Autodesk Fusion 360 part; units mm, degrees
(part 10 of 24)
  arc A1593 (61.7791, 45.6255) -> (62.0966, 45.6255) centre (61.9379, 45.6255) ccw
  arc A1594 (67.3925, 42.1213) -> (67.71, 42.1213) centre (67.5513, 42.1213) ccw
  arc A1595 (61.9357, 46.3347) -> (61.6424, 46.2132) centre (61.7891, 46.2739) ccw
  arc A1596 (63.9119, 46.0318) -> (63.7904, 45.7384) centre (63.8512, 45.8851) ccw
  line L433 (65.0555, 45.2726) -> (64.9496, 45.1667)
  arc A1597 (66.04, 45.4723) -> (66.04, 45.7898) centre (66.04, 45.6311) ccw
  line L434 (63.8511, 45.8851) -> (63.1489, 45.8851)
  line L435 (67.0245, 45.2726) -> (66.8321, 45.4124)
  line L436 (60.2439, 47.819) -> (59.8845, 47.9679)
  line L437 (66.04, 43.18) -> (67.5513, 43.18)
  arc A1598 (64.8373, 45.279) -> (65.0619, 45.0544) centre (64.9496, 45.1667) ccw
  line L438 (63.1489, 45.8851) -> (62.5, 45.6163)
  arc A1599 (65.6613, 45.7507) -> (65.7109, 45.4371) centre (65.6861, 45.5939) ccw
  arc A1600 (64.4392, 45.4697) -> (64.5607, 45.763) centre (64.4999, 45.6163) ccw
  arc A1601 (66.04, 43.3388) -> (66.04, 43.0213) centre (66.04, 43.1801) ccw
  line L439 (67.4406, 41.6601) -> (67.5141, 41.8863)
  arc A1602 (67.3573, 41.9111) -> (67.6709, 41.8615) centre (67.5141, 41.8863) ccw
  line L440 (67.5513, 42.1213) -> (67.5513, 43.18)
  line L441 (67.1928, 45.1043) -> (67.0245, 45.2726)
  line L442 (61.789, 46.2739) -> (60.519, 47.5439)
  arc A1603 (60.4068, 47.4317) -> (60.6313, 47.6562) centre (60.5191, 47.544) ccw
  arc A1604 (64.8373, 45.0544) -> (65.0619, 45.279) centre (64.9496, 45.1667) ccw
  arc A1605 (60.3562, 47.9313) -> (60.1317, 47.7068) centre (60.2439, 47.8191) ccw
  line L443 (65.2479, 45.4124) -> (65.0555, 45.2726)
  line L444 (64.9496, 45.1667) -> (64.5, 45.6163)
  arc A1606 (65.5319, 45.3789) -> (65.3878, 45.6618) centre (65.4599, 45.5204) ccw
  line L445 (67.0245, 41.0874) -> (67.1928, 41.2557)
  arc A1607 (66.5481, 40.9811) -> (66.6922, 40.6982) centre (66.6202, 40.8396) ccw
  arc A1608 (62.0966, 45.9145) -> (61.7791, 45.9145) centre (61.9379, 45.9145) ccw
  arc A1609 (67.3212, 45.1977) -> (67.0643, 45.011) centre (67.1928, 45.1044) ccw
  arc A1610 (59.9453, 48.1146) -> (59.8238, 47.8212) centre (59.8846, 47.9679) ccw
  line L446 (59.8845, 47.9679) -> (59.2617, 47.9679)
  arc A1611 (66.6922, 45.6618) -> (66.5481, 45.3789) centre (66.6201, 45.5204) ccw
  arc A1612 (60.1832, 47.6724) -> (60.3047, 47.9657) centre (60.2439, 47.8191) ccw
  arc A1613 (65.8813, 43.18) -> (66.1988, 43.18) centre (66.0401, 43.18) ccw
  arc A1614 (65.1677, 45.1603) -> (64.9432, 45.3848) centre (65.0555, 45.2726) ccw
  line L447 (60.519, 47.5439) -> (60.2439, 47.819)
  arc A1615 (61.8992, 45.4697) -> (62.0207, 45.763) centre (61.96, 45.6163) ccw
  line L448 (62.23, 45.3463) -> (61.96, 45.6163)
  arc A1616 (62.4393, 45.763) -> (62.5608, 45.4697) centre (62.5001, 45.6164) ccw
  line L449 (65.4599, 45.5204) -> (65.2479, 45.4124)
  arc A1617 (65.4108, 45.6714) -> (65.5089, 45.3694) centre (65.4598, 45.5204) ccw
  arc A1618 (61.7912, 45.8538) -> (62.0846, 45.9753) centre (61.9379, 45.9145) ccw
  arc A1619 (67.7081, 42.0964) -> (67.3945, 42.1461) centre (67.5513, 42.1212) ccw
  arc A1620 (64.9621, 45.401) -> (65.1488, 45.1441) centre (65.0555, 45.2726) ccw
  arc A1621 (67.3631, 44.4246) -> (67.6651, 44.5228) centre (67.5141, 44.4737) ccw
  line L450 (66.8321, 40.9476) -> (67.0245, 41.0874)
  arc A1622 (66.04, 43.0213) -> (66.04, 43.3388) centre (66.04, 43.1801) ccw
  arc A1623 (65.1758, 45.5538) -> (65.32, 45.2709) centre (65.2479, 45.4124) ccw
  line L451 (65.6861, 45.5939) -> (65.4599, 45.5204)
  arc A1624 (67.1368, 45.3848) -> (66.9123, 45.1603) centre (67.0246, 45.2726) ccw
  arc A1625 (63.8511, 45.7263) -> (63.8511, 46.0438) centre (63.8511, 45.8851) ccw
  arc A1626 (67.5513, 43.0212) -> (67.5513, 43.3387) centre (67.5513, 43.18) ccw
  arc A1627 (66.1987, 45.6311) -> (65.8812, 45.6311) centre (66.04, 45.6311) ccw
  line L452 (60.6089, 47.7647) -> (61.3111, 47.7647)
  arc A1628 (62.872, 49.1181) -> (62.5786, 49.2396) centre (62.7253, 49.1788) ccw
  line L453 (61.9379, 45.6255) -> (61.9379, 45.9145)
  line L454 (61.9379, 45.9145) -> (61.789, 46.2739)
  arc A1629 (65.8812, 43.18) -> (66.1987, 43.18) centre (66.04, 43.18) ccw
  line L455 (66.04, 45.6311) -> (65.9211, 45.6311)
  arc A1630 (58.8319, 51.442) -> (58.7104, 51.1486) centre (58.7711, 51.2953) ccw
  arc A1631 (57.3593, 51.1732) -> (57.4808, 50.8799) centre (57.42, 51.0266) ccw
  line L456 (61.3111, 51.2953) -> (60.6089, 51.2953)
  line L457 (61.3111, 47.7647) -> (61.96, 48.0335)
  arc A1632 (61.8477, 48.1457) -> (62.0722, 47.9212) centre (61.9599, 48.0335) ccw
  arc A1633 (62.5786, 49.8204) -> (62.872, 49.9419) centre (62.7253, 49.8812) ccw
  arc A1634 (65.7352, 45.4429) -> (65.637, 45.7449) centre (65.6861, 45.5939) ccw
  arc A1635 (59.5777, 50.8688) -> (59.8023, 50.6443) centre (59.69, 50.7566) ccw
  arc A1636 (62.0207, 47.8868) -> (61.8992, 48.1801) centre (61.9599, 48.0334) ccw
  arc A1637 (62.6032, 50.5907) -> (62.3099, 50.4692) centre (62.4566, 50.5299) ccw
  line L458 (61.96, 48.0335) -> (62.4565, 48.53)
  line L459 (66.04, 45.6311) -> (66.04, 43.18)
  arc A1638 (65.3412, 45.2839) -> (65.1546, 45.5408) centre (65.2479, 45.4124) ccw
  line L460 (57.15, 50.7565) -> (56.88, 51.0265)
  arc A1639 (62.5665, 49.1789) -> (62.884, 49.1789) centre (62.7253, 49.1789) ccw
  arc A1640 (60.0208, 48.1801) -> (59.8993, 47.8868) centre (59.96, 48.0335) ccw
  arc A1641 (59.8023, 48.1912) -> (59.5777, 48.4157) centre (59.69, 48.3035) ccw
  line L461 (59.2617, 47.9679) -> (59.42, 48.0335)
  arc A1642 (62.0722, 45.7286) -> (61.8477, 45.5041) centre (61.9599, 45.6164) ccw
  line L462 (61.96, 45.6163) -> (61.9379, 45.6255)
  line L463 (66.04, 43.18) -> (66.04, 45.6311)
  arc A1643 (59.5322, 51.1388) -> (59.3077, 50.9143) centre (59.42, 51.0266) ccw
  arc A1644 (59.8478, 47.9212) -> (60.0723, 48.1457) centre (59.9601, 48.0334) ccw
  arc A1645 (60.6313, 47.6562) -> (60.4068, 47.4317) centre (60.5191, 47.5439) ccw
  arc A1646 (59.3077, 48.1457) -> (59.5322, 47.9212) centre (59.42, 48.0335) ccw
  arc A1647 (62.1177, 45.2341) -> (62.3423, 45.4586) centre (62.23, 45.3464) ccw
  arc A1648 (61.6768, 46.1617) -> (61.9013, 46.3862) centre (61.7891, 46.2739) ccw
  arc A1649 (60.6089, 47.9235) -> (60.6089, 47.606) centre (60.6089, 47.7648) ccw
  line L464 (58.7711, 51.2953) -> (58.0689, 51.2953)
  arc A1650 (57.5323, 50.9143) -> (57.3078, 51.1388) centre (57.4201, 51.0266) ccw
  line L465 (62.5, 45.6163) -> (62.23, 45.3463)
  arc A1651 (65.9211, 45.7898) -> (65.9211, 45.4723) centre (65.9211, 45.6311) ccw
  arc A1652 (59.8845, 47.8091) -> (59.8845, 48.1266) centre (59.8845, 47.9679) ccw
  arc A1653 (59.3592, 50.8799) -> (59.4807, 51.1732) centre (59.42, 51.0266) ccw
  arc A1654 (58.1296, 51.1486) -> (58.0081, 51.442) centre (58.0689, 51.2953) ccw
  arc A1655 (62.0722, 51.1388) -> (61.8477, 50.9143) centre (61.9599, 51.0266) ccw
  arc A1656 (66.1589, 45.4723) -> (66.1589, 45.7898) centre (66.1589, 45.6311) ccw
  line L466 (59.69, 50.7565) -> (59.42, 51.0265)
  line L467 (62.7253, 49.1789) -> (62.7253, 49.8811)
  arc A1657 (56.9922, 51.1388) -> (56.7677, 50.9143) centre (56.88, 51.0266) ccw
  arc A1658 (63.2096, 45.7384) -> (63.0881, 46.0318) centre (63.1488, 45.8851) ccw
  arc A1659 (60.5481, 47.618) -> (60.6696, 47.9114) centre (60.6089, 47.7647) ccw
  arc A1660 (64.6122, 45.7286) -> (64.3877, 45.5041) centre (64.4999, 45.6163) ccw
  arc A1661 (62.5688, 48.4178) -> (62.3443, 48.6423) centre (62.4565, 48.53) ccw
  arc A1662 (62.1177, 45.4586) -> (62.3423, 45.2341) centre (62.23, 45.3464) ccw
  arc A1663 (65.8813, 43.18) -> (66.1988, 43.18) centre (66.0401, 43.18) ccw
  line L468 (57.42, 51.0265) -> (57.15, 50.7565)
  arc A1664 (57.0377, 50.8688) -> (57.2623, 50.6443) centre (57.15, 50.7566) ccw
  arc A1665 (66.04, 43.3388) -> (66.04, 43.0213) centre (66.04, 43.1801) ccw
  arc A1666 (61.3111, 51.1365) -> (61.3111, 51.454) centre (61.3111, 51.2953) ccw
  arc A1667 (61.2504, 47.9114) -> (61.3719, 47.618) centre (61.3111, 47.7647) ccw
  line L469 (62.4565, 50.53) -> (61.96, 51.0265)
  arc A1668 (59.5777, 50.6443) -> (59.8023, 50.8688) centre (59.69, 50.7566) ccw
  line L470 (62.7253, 49.8811) -> (62.4565, 50.53)
  arc A1669 (60.6089, 51.454) -> (60.6089, 51.1365) centre (60.6089, 51.2953) ccw
  arc A1670 (58.0689, 51.454) -> (58.0689, 51.1365) centre (58.0689, 51.2953) ccw
  line L471 (58.0689, 51.2953) -> (57.42, 51.0265)
  line L472 (59.42, 48.0335) -> (59.69, 48.3035)
  line L473 (51.1511, 51.2953) -> (50.4489, 51.2953)
  arc A1671 (57.0377, 50.6443) -> (57.2623, 50.8688) centre (57.15, 50.7566) ccw
  arc A1672 (49.7393, 51.1732) -> (49.8608, 50.8799) centre (49.8, 51.0266) ccw
  arc A1673 (49.1992, 50.8799) -> (49.3207, 51.1732) centre (49.26, 51.0266) ccw
  arc A1674 (52.9889, 51.454) -> (52.9889, 51.1365) centre (52.9889, 51.2953) ccw
  line L474 (59.96, 51.0265) -> (59.69, 50.7565)
  arc A1675 (52.4523, 50.9143) -> (52.2278, 51.1388) centre (52.34, 51.0266) ccw
  arc A1676 (61.3111, 47.606) -> (61.3111, 47.9235) centre (61.3111, 47.7648) ccw
  arc A1677 (59.2617, 48.1266) -> (59.2617, 47.8091) centre (59.2617, 47.9679) ccw
  arc A1678 (59.4807, 47.8868) -> (59.3592, 48.1801) centre (59.42, 48.0335) ccw
  arc A1679 (59.8993, 51.1732) -> (60.0208, 50.8799) centre (59.9601, 51.0266) ccw
  line L475 (59.96, 48.0335) -> (60.6089, 47.7647)
  arc A1680 (61.8992, 50.8799) -> (62.0207, 51.1732) centre (61.9599, 51.0266) ccw
  line L476 (59.42, 51.0265) -> (58.7711, 51.2953)
  line L477 (52.9889, 51.2953) -> (52.34, 51.0265)
  line L478 (49.8, 51.0265) -> (49.53, 50.7565)
  line L479 (61.96, 51.0265) -> (61.3111, 51.2953)
  arc A1681 (47.9089, 51.454) -> (47.9089, 51.1365) centre (47.9089, 51.2953) ccw
  arc A1682 (55.5289, 51.454) -> (55.5289, 51.1365) centre (55.5289, 51.2953) ccw
  arc A1683 (62.884, 49.8811) -> (62.5665, 49.8811) centre (62.7253, 49.8811) ccw
  arc A1684 (51.9122, 51.1388) -> (51.6877, 50.9143) centre (51.7999, 51.0266) ccw
  line L480 (54.34, 51.0265) -> (53.6911, 51.2953)
  arc A1685 (54.2792, 50.8799) -> (54.4007, 51.1732) centre (54.34, 51.0266) ccw
  arc A1686 (61.3719, 51.442) -> (61.2504, 51.1486) centre (61.3112, 51.2953) ccw
  line L481 (60.6089, 51.2953) -> (59.96, 51.0265)
  arc A1687 (46.8322, 51.1388) -> (46.6077, 50.9143) centre (46.72, 51.0266) ccw
  arc A1688 (54.4977, 50.8688) -> (54.7223, 50.6443) centre (54.61, 50.7566) ccw
  arc A1689 (51.1511, 51.1365) -> (51.1511, 51.454) centre (51.1511, 51.2953) ccw
  arc A1690 (52.2793, 51.1732) -> (52.4008, 50.8799) centre (52.3401, 51.0266) ccw
  line L482 (56.2311, 51.2953) -> (55.5289, 51.2953)
  line L483 (54.61, 50.7565) -> (54.34, 51.0265)
  arc A1691 (46.6592, 50.8799) -> (46.7807, 51.1732) centre (46.72, 51.0265) ccw
  arc A1692 (47.3723, 50.9143) -> (47.1478, 51.1388) centre (47.2601, 51.0266) ccw
  line L484 (51.8, 51.0265) -> (51.1511, 51.2953)
  arc A1693 (54.4522, 51.1388) -> (54.2277, 50.9143) centre (54.3399, 51.0266) ccw
  line L485 (50.4489, 51.2953) -> (49.8, 51.0265)
  arc A1694 (46.8777, 50.8688) -> (47.1023, 50.6443) centre (46.99, 50.7566) ccw
  arc A1695 (46.8777, 50.6443) -> (47.1023, 50.8688) centre (46.99, 50.7566) ccw
  arc A1696 (56.2919, 51.442) -> (56.1704, 51.1486) centre (56.2311, 51.2953) ccw
  line L486 (59.69, 48.3035) -> (59.96, 48.0335)
  arc A1697 (59.2009, 48.1146) -> (59.3224, 47.8212) centre (59.2616, 47.9679) ccw
  arc A1698 (58.7711, 51.1365) -> (58.7711, 51.454) centre (58.7711, 51.2953) ccw
  line L487 (49.53, 50.7565) -> (49.26, 51.0265)
  line L488 (46.72, 51.0265) -> (46.0711, 51.2953)
  line L489 (49.26, 51.0265) -> (48.6111, 51.2953)
  arc A1699 (54.4977, 50.6443) -> (54.7223, 50.8688) centre (54.61, 50.7566) ccw
  arc A1700 (60.0723, 50.9143) -> (59.8478, 51.1388) centre (59.9601, 51.0266) ccw
  line L490 (53.6911, 51.2953) -> (52.9889, 51.2953)
  arc A1701 (62.3099, 48.5908) -> (62.6032, 48.4693) centre (62.4566, 48.5301) ccw
  arc A1702 (54.8193, 51.1732) -> (54.9408, 50.8799) centre (54.8801, 51.0266) ccw
  arc A1703 (46.1319, 51.442) -> (46.0104, 51.1486) centre (46.0712, 51.2953) ccw
  arc A1704 (56.2311, 51.1365) -> (56.2311, 51.454) centre (56.2311, 51.2953) ccw
  line L491 (62.4565, 48.53) -> (62.7253, 49.1789)
  arc A1705 (54.9923, 50.9143) -> (54.7678, 51.1388) centre (54.8801, 51.0266) ccw
  arc A1706 (62.3443, 50.4177) -> (62.5688, 50.6422) centre (62.4566, 50.53) ccw
  line L492 (46.99, 50.7565) -> (46.72, 51.0265)
  line L493 (47.9089, 51.2953) -> (47.26, 51.0265)
  arc A1707 (55.5896, 51.1486) -> (55.4681, 51.442) centre (55.5289, 51.2953) ccw
  arc A1708 (51.2119, 51.442) -> (51.0904, 51.1486) centre (51.1512, 51.2953) ccw
  arc A1709 (50.4489, 51.454) -> (50.4489, 51.1365) centre (50.4489, 51.2953) ccw
  arc A1710 (60.6696, 51.1486) -> (60.5481, 51.442) centre (60.6089, 51.2953) ccw
  arc A1711 (59.8023, 48.4157) -> (59.5777, 48.1912) centre (59.69, 48.3035) ccw
  arc A1712 (51.9577, 50.6443) -> (52.1823, 50.8688) centre (52.07, 50.7566) ccw
  arc A1713 (53.7519, 51.442) -> (53.6304, 51.1486) centre (53.6912, 51.2953) ccw
  arc A1714 (42.2923, 50.9143) -> (42.0678, 51.1388) centre (42.18, 51.0266) ccw
  line L494 (54.88, 51.0265) -> (54.61, 50.7565)
  arc A1715 (47.1993, 51.1732) -> (47.3208, 50.8799) centre (47.26, 51.0266) ccw
  arc A1716 (41.7977, 50.6443) -> (42.0223, 50.8688) centre (41.91, 50.7566) ccw
  arc A1717 (53.6911, 51.1365) -> (53.6911, 51.454) centre (53.6911, 51.2953) ccw
  line L495 (47.26, 51.0265) -> (46.99, 50.7565)
  arc A1718 (49.4177, 50.6443) -> (49.6423, 50.8688) centre (49.53, 50.7566) ccw
  line L496 (45.3689, 51.2953) -> (44.72, 51.0265)
  arc A1719 (51.7392, 50.8799) -> (51.8607, 51.1732) centre (51.7999, 51.0266) ccw
  line L497 (43.5311, 51.2953) -> (42.8289, 51.2953)
  arc A1720 (36.4992, 50.8799) -> (36.6207, 51.1732) centre (36.56, 51.0266) ccw
  arc A1721 (43.5311, 51.1365) -> (43.5311, 51.454) centre (43.5311, 51.2953) ccw
  line L498 (37.7489, 51.2953) -> (37.1, 51.0265)
  line L499 (35.9111, 51.2953) -> (35.2089, 51.2953)
  arc A1722 (37.0393, 51.1732) -> (37.1608, 50.8799) centre (37.1, 51.0266) ccw
  arc A1723 (37.2123, 50.9143) -> (36.9878, 51.1388) centre (37.1001, 51.0266) ccw
  arc A1724 (48.6719, 51.442) -> (48.5504, 51.1486) centre (48.6112, 51.2953) ccw
  arc A1725 (51.9577, 50.8688) -> (52.1823, 50.6443) centre (52.07, 50.7566) ccw
  line L500 (37.1, 51.0265) -> (36.83, 50.7565)
  line L501 (39.64, 51.0265) -> (39.37, 50.7565)
  arc A1726 (36.6722, 51.1388) -> (36.4477, 50.9143) centre (36.56, 51.0266) ccw
  line L502 (55.5289, 51.2953) -> (54.88, 51.0265)
  arc A1727 (38.5119, 51.442) -> (38.3904, 51.1486) centre (38.4511, 51.2953) ccw
  arc A1728 (35.9719, 51.442) -> (35.8504, 51.1486) centre (35.9112, 51.2953) ccw
  line L503 (56.88, 51.0265) -> (56.2311, 51.2953)
  arc A1729 (50.5096, 51.1486) -> (50.3881, 51.442) centre (50.4489, 51.2953) ccw
  arc A1730 (49.3722, 51.1388) -> (49.1477, 50.9143) centre (49.26, 51.0266) ccw
  arc A1731 (56.8192, 50.8799) -> (56.9407, 51.1732) centre (56.88, 51.0266) ccw
  arc A1732 (47.9696, 51.1486) -> (47.8481, 51.442) centre (47.9089, 51.2953) ccw
  arc A1733 (36.7177, 50.8688) -> (36.9423, 50.6443) centre (36.83, 50.7566) ccw
  line L504 (48.6111, 51.2953) -> (47.9089, 51.2953)
  line L505 (36.83, 50.7565) -> (36.56, 51.0265)
  line L506 (46.0711, 51.2953) -> (45.3689, 51.2953)
  line L507 (44.72, 51.0265) -> (44.45, 50.7565)
  arc A1734 (41.7522, 51.1388) -> (41.5277, 50.9143) centre (41.6399, 51.0266) ccw
  arc A1735 (38.4511, 51.1365) -> (38.4511, 51.454) centre (38.4511, 51.2953) ccw
  arc A1736 (37.8096, 51.1486) -> (37.6881, 51.442) centre (37.7489, 51.2953) ccw
  arc A1737 (53.0496, 51.1486) -> (52.9281, 51.442) centre (52.9888, 51.2953) ccw
  line L508 (52.07, 50.7565) -> (51.8, 51.0265)
  arc A1738 (36.7177, 50.6443) -> (36.9423, 50.8688) centre (36.83, 50.7566) ccw
  arc A1739 (44.3377, 50.6443) -> (44.5623, 50.8688) centre (44.45, 50.7566) ccw
  line L509 (41.91, 50.7565) -> (41.64, 51.0265)
  arc A1740 (35.2089, 51.454) -> (35.2089, 51.1365) centre (35.2089, 51.2953) ccw
  arc A1741 (44.3377, 50.8688) -> (44.5623, 50.6443) centre (44.45, 50.7566) ccw
  arc A1742 (45.3689, 51.454) -> (45.3689, 51.1365) centre (45.3689, 51.2953) ccw
  arc A1743 (48.6111, 51.1365) -> (48.6111, 51.454) centre (48.6111, 51.2953) ccw
  arc A1744 (39.0392, 50.8799) -> (39.1607, 51.1732) centre (39.1, 51.0266) ccw
  arc A1745 (44.1192, 50.8799) -> (44.2407, 51.1732) centre (44.1799, 51.0266) ccw
  line L510 (42.8289, 51.2953) -> (42.18, 51.0265)
  line L511 (39.1, 51.0265) -> (38.4511, 51.2953)
  line L512 (35.2089, 51.2953) -> (34.56, 51.0265)
  arc A1746 (44.8323, 50.9143) -> (44.6078, 51.1388) centre (44.72, 51.0266) ccw
  arc A1747 (49.4177, 50.8688) -> (49.6423, 50.6443) centre (49.53, 50.7566) ccw
  arc A1748 (49.9123, 50.9143) -> (49.6878, 51.1388) centre (49.8, 51.0266) ccw
  arc A1749 (39.2577, 50.8688) -> (39.4823, 50.6443) centre (39.37, 50.7566) ccw
  line L513 (36.56, 51.0265) -> (35.9111, 51.2953)
  arc A1750 (42.8896, 51.1486) -> (42.7681, 51.442) centre (42.8289, 51.2953) ccw
  arc A1751 (44.6593, 51.1732) -> (44.7808, 50.8799) centre (44.7201, 51.0266) ccw
  arc A1752 (35.9111, 51.1365) -> (35.9111, 51.454) centre (35.9111, 51.2953) ccw
  arc A1753 (42.1193, 51.1732) -> (42.2408, 50.8799) centre (42.1801, 51.0266) ccw
  arc A1754 (41.0519, 51.442) -> (40.9304, 51.1486) centre (40.9912, 51.2953) ccw
  line L514 (52.34, 51.0265) -> (52.07, 50.7565)
  line L515 (44.45, 50.7565) -> (44.18, 51.0265)
  line L516 (38.4511, 51.2953) -> (37.7489, 51.2953)
  arc A1755 (31.5768, 50.795) -> (31.3523, 50.5705) centre (31.4645, 50.6827) ccw
  arc A1756 (30.48, 51.2) -> (30.48, 50.8825) centre (30.48, 51.0413) ccw
  arc A1757 (30.6238, 51.1981) -> (30.5741, 50.8845) centre (30.599, 51.0413) ccw
  arc A1758 (29.7812, 50.6941) -> (29.5946, 50.951) centre (29.6879, 50.8225) ccw
  arc A1759 (42.8289, 51.454) -> (42.8289, 51.1365) centre (42.8289, 51.2953) ccw
  arc A1760 (30.1752, 50.8531) -> (30.077, 51.1551) centre (30.1261, 51.0041) ccw
  arc A1761 (40.9911, 51.1365) -> (40.9911, 51.454) centre (40.9911, 51.2953) ccw
  arc A1762 (39.7523, 50.9143) -> (39.5278, 51.1388) centre (39.64, 51.0266) ccw
  arc A1763 (31.2, 50.6811) -> (31.3442, 50.964) centre (31.2721, 50.8226) ccw
  arc A1764 (32.7296, 51.1486) -> (32.6081, 51.442) centre (32.6689, 51.2953) ccw
  line L517 (31.5704, 50.5769) -> (31.4645, 50.6828)
  arc A1765 (30.5989, 50.8825) -> (30.5989, 51.2) centre (30.5989, 51.0413) ccw
  arc A1766 (30.48, 49.3713) -> (30.48, 49.6888) centre (30.48, 49.5301) ccw
  line L518 (32.6689, 51.2953) -> (32.02, 51.0265)
  line L519 (29.6879, 50.8226) -> (29.4955, 50.6828)
  arc A1767 (34.1322, 51.1388) -> (33.9077, 50.9143) centre (34.0199, 51.0266) ccw
  line L520 (31.4645, 50.6828) -> (31.2721, 50.8226)
  line L521 (31.2721, 50.8226) -> (31.0601, 50.9306)
  arc A1768 (29.215, 50.6268) -> (29.4395, 50.4023) centre (29.3273, 50.5146) ccw
  arc A1769 (30.8091, 50.8473) -> (30.8587, 51.1609) centre (30.8339, 51.0041) ccw
  line L522 (30.5989, 51.0413) -> (30.48, 51.0413)
  arc A1770 (32.1323, 50.9143) -> (31.9078, 51.1388) centre (32.0201, 51.0266) ccw
  arc A1771 (30.3213, 49.53) -> (30.6388, 49.53) centre (30.4801, 49.53) ccw
  arc A1772 (31.0111, 50.7796) -> (31.1092, 51.0816) centre (31.0602, 50.9306) ccw
  line L523 (29.4955, 50.6828) -> (29.3272, 50.5145)
  arc A1773 (29.4021, 50.8112) -> (29.5888, 50.5543) centre (29.4955, 50.6827) ccw
  line L524 (34.56, 51.0265) -> (34.29, 50.7565)
  line L525 (39.37, 50.7565) -> (39.1, 51.0265)
  arc A1774 (34.4993, 51.1732) -> (34.6208, 50.8799) centre (34.5601, 51.0266) ccw
  line L526 (30.3611, 51.0413) -> (30.1261, 51.0041)
  arc A1775 (29.9719, 50.7891) -> (29.8278, 51.072) centre (29.8999, 50.9306) ccw
  arc A1776 (40.2889, 51.454) -> (40.2889, 51.1365) centre (40.2889, 51.2953) ccw
  arc A1777 (31.4581, 50.6892) -> (31.6826, 50.4646) centre (31.5704, 50.5769) ccw
  arc A1778 (41.7977, 50.8688) -> (42.0223, 50.6443) centre (41.91, 50.7566) ccw
  line L527 (40.2889, 51.2953) -> (39.64, 51.0265)
  arc A1779 (37.7489, 51.454) -> (37.7489, 51.1365) centre (37.7489, 51.2953) ccw
  arc A1780 (39.2577, 50.6443) -> (39.4823, 50.8688) centre (39.37, 50.7566) ccw
  arc A1781 (31.9593, 51.1732) -> (32.0808, 50.8799) centre (32.0201, 51.0266) ccw
  line L528 (30.8339, 51.0041) -> (30.5989, 51.0413)
  arc A1782 (30.883, 51.1551) -> (30.7848, 50.8531) centre (30.8339, 51.0041) ccw
  arc A1783 (29.6158, 50.964) -> (29.76, 50.6811) centre (29.6879, 50.8225) ccw
  line L529 (41.64, 51.0265) -> (40.9911, 51.2953)
  arc A1784 (30.6388, 51.0413) -> (30.3213, 51.0413) centre (30.4801, 51.0413) ccw
  line L530 (34.29, 50.7565) -> (34.02, 51.0265)
  line L531 (42.18, 51.0265) -> (41.91, 50.7565)
  arc A1785 (31.3654, 50.951) -> (31.1788, 50.6941) centre (31.2721, 50.8225) ccw
  line L532 (30.48, 51.0413) -> (30.3611, 51.0413)
  arc A1786 (39.5793, 51.1732) -> (39.7008, 50.8799) centre (39.6401, 51.0266) ccw
  arc A1787 (46.0711, 51.1365) -> (46.0711, 51.454) centre (46.0711, 51.2953) ccw
  arc A1788 (30.3611, 51.2) -> (30.3611, 50.8825) centre (30.3611, 51.0413) ccw
  line L533 (44.18, 51.0265) -> (43.5311, 51.2953)
  line L534 (40.9911, 51.2953) -> (40.2889, 51.2953)
  arc A1789 (43.5919, 51.442) -> (43.4704, 51.1486) centre (43.5312, 51.2953) ccw
  arc A1790 (40.3496, 51.1486) -> (40.2281, 51.442) centre (40.2889, 51.2953) ccw
  line L535 (30.48, 49.53) -> (30.48, 51.0413)
  arc A1791 (29.6077, 50.5705) -> (29.3832, 50.795) centre (29.4954, 50.6827) ccw
  arc A1792 (41.5792, 50.8799) -> (41.7007, 51.1732) centre (41.6399, 51.0266) ccw
  arc A1793 (35.2696, 51.1486) -> (35.1481, 51.442) centre (35.2089, 51.2953) ccw
  arc A1794 (39.2122, 51.1388) -> (38.9877, 50.9143) centre (39.1, 51.0266) ccw
  arc A1795 (33.4319, 51.442) -> (33.3104, 51.1486) centre (33.3712, 51.2953) ccw
  arc A1796 (45.4296, 51.1486) -> (45.3081, 51.442) centre (45.3689, 51.2953) ccw
  arc A1797 (44.2922, 51.1388) -> (44.0677, 50.9143) centre (44.1799, 51.0266) ccw
  arc A1798 (34.1777, 50.6443) -> (34.4023, 50.8688) centre (34.29, 50.7565) ccw
  arc A1799 (33.3711, 51.1365) -> (33.3711, 51.454) centre (33.3711, 51.2953) ccw
  arc A1800 (26.7373, 50.4646) -> (26.9619, 50.6892) centre (26.8496, 50.5769) ccw
  arc A1801 (27.6352, 50.8531) -> (27.537, 51.1551) centre (27.5861, 51.0041) ccw
  arc A1802 (27.94, 49.3713) -> (27.94, 49.6888) centre (27.94, 49.5301) ccw
  arc A1803 (30.3859, 50.8845) -> (30.3362, 51.1981) centre (30.361, 51.0413) ccw
  line L536 (27.94, 51.0413) -> (27.8211, 51.0413)
  line L537 (32.02, 51.0265) -> (31.5704, 50.5769)
  arc A1804 (30.48, 49.6888) -> (30.48, 49.3713) centre (30.48, 49.5301) ccw
  line L538 (29.0928, 50.5145) -> (28.9245, 50.6828)
  arc A1805 (25.8119, 51.442) -> (25.6904, 51.1486) centre (25.7512, 51.2953) ccw
  arc A1806 (27.2412, 50.6941) -> (27.0546, 50.951) centre (27.1479, 50.8225) ccw
  arc A1807 (26.3392, 50.8799) -> (26.4607, 51.1732) centre (26.3999, 51.0266) ccw
  line L539 (25.7511, 51.2953) -> (25.0489, 51.2953)
  arc A1808 (32.6689, 51.454) -> (32.6689, 51.1365) centre (32.6689, 51.2953) ccw
  arc A1809 (25.0489, 51.454) -> (25.0489, 51.1365) centre (25.0489, 51.2953) ccw
  arc A1810 (23.9342, 50.7853) -> (24.1587, 50.5607) centre (24.0465, 50.673) ccw
  arc A1811 (28.66, 50.6811) -> (28.8042, 50.964) centre (28.7321, 50.8226) ccw
  arc A1812 (26.8621, 50.8112) -> (27.0488, 50.5543) centre (26.9554, 50.6827) ccw
  line L540 (31.0601, 50.9306) -> (30.8339, 51.0041)
  arc A1813 (29.8508, 51.0816) -> (29.9489, 50.7796) centre (29.8999, 50.9306) ccw
  line L541 (26.8496, 50.5769) -> (26.4, 51.0265)
  arc A1814 (29.0816, 50.2599) -> (29.3384, 50.4465) centre (29.21, 50.3532) ccw
  line L542 (25.0489, 51.2953) -> (24.4, 51.0265)
  arc A1815 (27.7813, 49.53) -> (28.0988, 49.53) centre (27.9401, 49.53) ccw
  line L543 (27.94, 49.53) -> (27.94, 51.0413)
  arc A1816 (34.1777, 50.8688) -> (34.4023, 50.6443) centre (34.29, 50.7566) ccw
  arc A1817 (30.6387, 51.0413) -> (30.3212, 51.0413) centre (30.48, 51.0413) ccw
  arc A1818 (30.3212, 49.53) -> (30.6387, 49.53) centre (30.48, 49.53) ccw
  arc A1819 (30.1013, 51.1609) -> (30.1509, 50.8473) centre (30.1261, 51.0041) ccw
  arc A1820 (27.0677, 50.5705) -> (26.8432, 50.795) centre (26.9554, 50.6827) ccw
  line L544 (27.94, 51.0413) -> (27.94, 49.53)
  arc A1821 (26.5122, 51.1388) -> (26.2877, 50.9143) centre (26.3999, 51.0266) ccw
  line L545 (27.5861, 51.0041) -> (27.3599, 50.9306)
  arc A1822 (28.0838, 51.1981) -> (28.0341, 50.8845) centre (28.0589, 51.0413) ccw
  line L546 (24.4, 51.0265) -> (24.0465, 50.673)
  arc A1823 (28.9805, 50.4023) -> (29.205, 50.6268) centre (29.0928, 50.5146) ccw
  line L547 (26.4, 51.0265) -> (25.7511, 51.2953)
  arc A1824 (31.4581, 50.4646) -> (31.6826, 50.6892) centre (31.5704, 50.5769) ccw
  arc A1825 (34.6723, 50.9143) -> (34.4478, 51.1388) centre (34.5601, 51.0266) ccw
  arc A1826 (24.3393, 51.1732) -> (24.4608, 50.8799) centre (24.4001, 51.0266) ccw
  line L548 (33.3711, 51.2953) -> (32.6689, 51.2953)
  arc A1827 (26.7373, 50.6892) -> (26.9619, 50.4646) centre (26.8496, 50.5769) ccw
  arc A1828 (25.1096, 51.1486) -> (24.9881, 51.442) centre (25.0489, 51.2953) ccw
  arc A1829 (31.1322, 51.072) -> (30.9881, 50.7891) centre (31.0602, 50.9306) ccw
  arc A1830 (27.0758, 50.964) -> (27.22, 50.6811) centre (27.1479, 50.8225) ccw
  arc A1831 (31.3712, 50.5543) -> (31.5579, 50.8112) centre (31.4646, 50.6827) ccw
  arc A1832 (27.4319, 50.7891) -> (27.2878, 51.072) centre (27.3599, 50.9306) ccw
  arc A1833 (28.5922, 51.072) -> (28.4481, 50.7891) centre (28.5202, 50.9306) ccw
  line L549 (28.9245, 50.6828) -> (28.7321, 50.8226)
  line L550 (26.9555, 50.6828) -> (26.8496, 50.5769)
  line L551 (28.2939, 51.0041) -> (28.0589, 51.0413)
  arc A1834 (27.94, 50.8825) -> (27.94, 51.2) centre (27.94, 51.0413) ccw
  line L552 (28.7321, 50.8226) -> (28.5201, 50.9306)
  arc A1835 (25.7511, 51.1365) -> (25.7511, 51.454) centre (25.7511, 51.2953) ccw
  arc A1836 (28.343, 51.1551) -> (28.2448, 50.8531) centre (28.2939, 51.0041) ccw
  line L553 (30.1261, 51.0041) -> (29.8999, 50.9306)
  arc A1837 (30.48, 50.8825) -> (30.48, 51.2) centre (30.48, 51.0413) ccw
  line L554 (30.48, 51.0413) -> (30.48, 49.53)
  arc A1838 (27.7812, 49.53) -> (28.0987, 49.53) centre (27.94, 49.53) ccw
  arc A1839 (28.8254, 50.951) -> (28.6388, 50.6941) centre (28.7321, 50.8225) ccw
  arc A1840 (29.0816, 50.4465) -> (29.3384, 50.2599) centre (29.21, 50.3532) ccw
  arc A1841 (33.9592, 50.8799) -> (34.0807, 51.1732) centre (34.02, 51.0266) ccw
  line L555 (29.8999, 50.9306) -> (29.6879, 50.8226)
  line L556 (34.02, 51.0265) -> (33.3711, 51.2953)
  arc A1842 (28.4711, 50.7796) -> (28.5692, 51.0816) centre (28.5202, 50.9306) ccw
  arc A1843 (19.2087, 51.9811) -> (18.8912, 51.9811) centre (19.05, 51.9811) ccw
  arc A1844 (22.0019, 52.3818) -> (21.8804, 52.0884) centre (21.9412, 52.2351) ccw
  line L557 (19.05, 49.53) -> (19.05, 51.9811)
  line L558 (23.3553, 50.8209) -> (23.0865, 51.4698)
  arc A1845 (18.4208, 52.0214) -> (18.5189, 51.7194) centre (18.4698, 51.8704) ccw
  arc A1846 (28.0987, 51.0413) -> (27.7812, 51.0413) centre (27.94, 51.0413) ccw
  arc A1847 (18.9559, 51.8243) -> (18.9062, 52.1379) centre (18.931, 51.9811) ccw
  line L559 (29.3272, 50.5145) -> (29.21, 50.3532)
  arc A1848 (23.3553, 50.8317) -> (23.3553, 50.5142) centre (23.3553, 50.673) ccw
  arc A1849 (28.0589, 50.8825) -> (28.0589, 51.2) centre (28.0589, 51.0413) ccw
  arc A1850 (29.0368, 50.795) -> (28.8123, 50.5705) centre (28.9245, 50.6827) ccw
  arc A1851 (29.2212, 50.6079) -> (28.9643, 50.4212) centre (29.0928, 50.5145) ccw
  arc A1852 (28.0988, 51.0413) -> (27.7813, 51.0413) centre (27.9401, 51.0413) ccw
  line L560 (23.3553, 50.673) -> (23.3553, 50.8209)
  arc A1853 (21.9411, 52.0763) -> (21.9411, 52.3938) centre (21.9411, 52.2351) ccw
  arc A1854 (20.7023, 51.8541) -> (20.4778, 52.0786) centre (20.5901, 51.9664) ccw
  arc A1855 (23.1965, 50.673) -> (23.514, 50.673) centre (23.3553, 50.673) ccw
  arc A1856 (19.05, 52.1398) -> (19.05, 51.8223) centre (19.05, 51.9811) ccw
  line L561 (20.0345, 51.6226) -> (19.8421, 51.7624)
  arc A1857 (27.8211, 51.2) -> (27.8211, 50.8825) centre (27.8211, 51.0413) ccw
  arc A1858 (19.05, 49.3713) -> (19.05, 49.6888) centre (19.05, 49.5301) ccw
  line L562 (21.9411, 52.2351) -> (21.2389, 52.2351)
  arc A1859 (21.2389, 52.3938) -> (21.2389, 52.0763) centre (21.2389, 52.2351) ccw
  arc A1860 (27.94, 51.2) -> (27.94, 50.8825) centre (27.94, 51.0413) ccw
  arc A1861 (27.94, 49.6888) -> (27.94, 49.3713) centre (27.94, 49.5301) ccw
  arc A1862 (20.5293, 52.113) -> (20.6508, 51.8197) centre (20.5901, 51.9664) ccw
  arc A1863 (20.1468, 51.7348) -> (19.9223, 51.5103) centre (20.0345, 51.6226) ccw
  arc A1864 (18.1858, 51.9038) -> (18.33, 51.6209) centre (18.2579, 51.7623) ccw
  arc A1865 (18.5419, 51.7289) -> (18.3978, 52.0118) centre (18.4699, 51.8704) ccw
  arc A1866 (20.0281, 51.629) -> (20.2526, 51.4044) centre (20.1404, 51.5167) ccw
  arc A1867 (19.5811, 51.7194) -> (19.6792, 52.0214) centre (19.6302, 51.8704) ccw
  line L563 (19.05, 51.9811) -> (19.05, 49.53)
  line L564 (19.1689, 51.9811) -> (19.05, 51.9811)
  arc A1868 (22.7022, 52.0786) -> (22.4777, 51.8541) centre (22.59, 51.9664) ccw
  line L565 (22.59, 51.9663) -> (21.9411, 52.2351)
  line L566 (19.6301, 51.8704) -> (19.4039, 51.9439)
  arc A1869 (27.3108, 51.0816) -> (27.4089, 50.7796) centre (27.3599, 50.9306) ccw
  arc A1870 (24.5123, 50.9143) -> (24.2878, 51.1388) centre (24.4001, 51.0266) ccw
  line L567 (24.0465, 50.673) -> (23.3553, 50.673)
  arc A1871 (28.2691, 50.8473) -> (28.3187, 51.1609) centre (28.2939, 51.0041) ccw
  line L568 (27.3599, 50.9306) -> (27.1479, 50.8226)
  line L569 (27.8211, 51.0413) -> (27.5861, 51.0041)
  line L570 (18.9311, 51.9811) -> (18.6961, 51.9439)
  arc A1872 (23.2332, 51.5305) -> (22.9399, 51.409) centre (23.0866, 51.4698) ccw
  arc A1873 (18.9311, 52.1398) -> (18.9311, 51.8223) centre (18.9311, 51.9811) ccw
  arc A1874 (21.2996, 52.0884) -> (21.1781, 52.3818) centre (21.2388, 52.2351) ccw
  arc A1875 (27.5613, 51.1609) -> (27.6109, 50.8473) centre (27.5861, 51.0041) ccw
  line L571 (19.8421, 51.7624) -> (19.6301, 51.8704)
  arc A1876 (27.8459, 50.8845) -> (27.7962, 51.1981) centre (27.821, 51.0413) ccw
  arc A1877 (18.7452, 51.7929) -> (18.647, 52.0949) centre (18.6961, 51.9439) ccw
  arc A1878 (19.9412, 51.4941) -> (20.1279, 51.751) centre (20.0346, 51.6226) ccw
  arc A1879 (19.05, 49.6888) -> (19.05, 49.3713) centre (19.05, 49.5301) ccw
  line L572 (28.5201, 50.9306) -> (28.2939, 51.0041)
  arc A1880 (29.4557, 50.4212) -> (29.1988, 50.6079) centre (29.3273, 50.5146) ccw
  line L573 (29.21, 50.3532) -> (29.0928, 50.5145)
  line L574 (18.6961, 51.9439) -> (18.4699, 51.8704)
  line L575 (18.4699, 51.8704) -> (18.2579, 51.7624)
  line L576 (18.2579, 51.7624) -> (18.0655, 51.6226)
  arc A1881 (23.514, 50.8209) -> (23.1965, 50.8209) centre (23.3553, 50.8209) ccw
  arc A1882 (22.5292, 51.8197) -> (22.6507, 52.113) centre (22.59, 51.9663) ccw
  line L577 (28.0589, 51.0413) -> (27.94, 51.0413)
  arc A1883 (28.8312, 50.5543) -> (29.0179, 50.8112) centre (28.9245, 50.6828) ccw
  line L578 (27.1479, 50.8226) -> (26.9555, 50.6828)
  line L579 (20.1404, 51.5167) -> (20.0345, 51.6226)
  arc A1884 (10.5423, 51.8541) -> (10.3178, 52.0786) centre (10.43, 51.9664) ccw
  line L580 (9.9335, 47.5902) -> (10.43, 47.0937)
  arc A1885 (10.0457, 47.7025) -> (9.8212, 47.478) centre (9.9335, 47.5903) ccw
  line L581 (10.43, 47.0937) -> (10.4521, 47.0845)
  line L582 (19.4039, 51.9439) -> (19.1689, 51.9811)
  arc A1886 (15.1277, 51.5841) -> (15.3523, 51.8086) centre (15.24, 51.6964) ccw
  arc A1887 (16.8611, 52.0763) -> (16.8611, 52.3938) centre (16.8611, 52.2351) ccw
  arc A1888 (18.6713, 52.1007) -> (18.7209, 51.7871) centre (18.6961, 51.9439) ccw
  arc A1889 (19.1938, 52.1379) -> (19.1441, 51.8243) centre (19.1689, 51.9811) ccw
  line L583 (21.2389, 52.2351) -> (20.59, 51.9663)
  line L584 (9.9335, 51.4698) -> (9.6647, 50.8209)
  line L585 (9.6647, 50.8209) -> (9.6647, 48.2391)
  arc A1890 (9.518, 50.8817) -> (9.8114, 50.7602) centre (9.6647, 50.821) ccw
  arc A1891 (16.1589, 52.3938) -> (16.1589, 52.0763) centre (16.1589, 52.2351) ccw
  arc A1892 (14.3211, 52.0763) -> (14.3211, 52.3938) centre (14.3211, 52.2351) ccw
  arc A1893 (10.3178, 46.9814) -> (10.5423, 47.2059) centre (10.43, 47.0936) ccw
  arc A1894 (19.7022, 52.0118) -> (19.5581, 51.7289) centre (19.6302, 51.8704) ccw
  arc A1895 (18.8912, 49.53) -> (19.2087, 49.53) centre (19.05, 49.53) ccw
  arc A1896 (18.3512, 51.6339) -> (18.1646, 51.8908) centre (18.2579, 51.7623) ccw
  arc A1897 (10.0801, 51.409) -> (9.7868, 51.5305) centre (9.9334, 51.4698) ccw
  line L586 (14.97, 51.9663) -> (14.3211, 52.2351)
  arc A1898 (24.0465, 50.5142) -> (24.0465, 50.8317) centre (24.0465, 50.673) ccw
  arc A1899 (9.8234, 50.8209) -> (9.506, 50.8209) centre (9.6647, 50.8209) ccw
  arc A1900 (10.3914, 46.9378) -> (10.5128, 47.2312) centre (10.4521, 47.0845) ccw
  arc A1901 (18.8913, 49.53) -> (19.2088, 49.53) centre (19.0501, 49.53) ccw
  line L587 (23.0865, 51.4698) -> (22.59, 51.9663)
  arc A1902 (19.3791, 51.7871) -> (19.4287, 52.1007) centre (19.4039, 51.9439) ccw
  arc A1903 (19.2088, 51.9811) -> (18.8913, 51.9811) centre (19.0501, 51.9811) ccw
  arc A1904 (23.2086, 50.7602) -> (23.502, 50.8817) centre (23.3553, 50.821) ccw
  arc A1905 (9.8114, 48.2998) -> (9.518, 48.1783) centre (9.6647, 48.239) ccw
  arc A1906 (19.9354, 51.8908) -> (19.7488, 51.6339) centre (19.8421, 51.7623) ccw
  line L588 (16.8611, 52.2351) -> (16.1589, 52.2351)
  arc A1907 (9.7868, 47.5295) -> (10.0801, 47.651) centre (9.9334, 47.5903) ccw
  arc A1908 (13.0823, 51.8541) -> (12.8578, 52.0786) centre (12.9701, 51.9664) ccw
  arc A1909 (13.6189, 52.3938) -> (13.6189, 52.0763) centre (13.6189, 52.2351) ccw
  line L589 (19.05, 51.9811) -> (18.9311, 51.9811)
  arc A1910 (11.1396, 52.0884) -> (11.0181, 52.3818) centre (11.0788, 52.2351) ccw
  arc A1911 (19.77, 51.6209) -> (19.9142, 51.9038) centre (19.8421, 51.7623) ccw
  arc A1912 (19.453, 52.0949) -> (19.3548, 51.7929) centre (19.4039, 51.9439) ccw
  line L590 (9.6647, 48.2391) -> (9.9335, 47.5902)
  arc A1913 (20.0281, 51.4044) -> (20.2526, 51.629) centre (20.1403, 51.5167) ccw
  arc A1914 (16.2196, 52.0884) -> (16.0981, 52.3818) centre (16.1589, 52.2351) ccw
  line L591 (15.24, 51.6963) -> (14.97, 51.9663)
  arc A1915 (12.3692, 51.8197) -> (12.4907, 52.113) centre (12.43, 51.9663) ccw
  arc A1916 (17.4492, 51.8197) -> (17.5707, 52.113) centre (17.51, 51.9663) ccw
  arc A1917 (22.9743, 51.3575) -> (23.1988, 51.582) centre (23.0865, 51.4698) ccw
  arc A1918 (9.8212, 51.582) -> (10.0457, 51.3575) centre (9.9335, 51.4698) ccw
  arc A1919 (11.8419, 52.3818) -> (11.7204, 52.0884) centre (11.7812, 52.2351) ccw
  line L592 (12.7, 51.6963) -> (12.43, 51.9663)
  arc A1920 (19.05, 51.8223) -> (19.05, 52.1398) centre (19.05, 51.9811) ccw
  arc A1921 (16.9219, 52.3818) -> (16.8004, 52.0884) centre (16.8612, 52.2351) ccw
  line L593 (10.43, 51.9663) -> (9.9335, 51.4698)
  line L594 (20.59, 51.9663) -> (20.1404, 51.5167)
  line L595 (18.0655, 51.6226) -> (17.9596, 51.5167)
  arc A1922 (9.506, 48.2391) -> (9.8234, 48.2391) centre (9.6647, 48.2391) ccw
  arc A1923 (17.9721, 51.751) -> (18.1588, 51.4941) centre (18.0654, 51.6226) ccw
  line L596 (17.51, 51.9663) -> (16.8611, 52.2351)
  arc A1924 (15.6223, 51.8541) -> (15.3978, 52.0786) centre (15.51, 51.9664) ccw
  arc A1925 (15.4493, 52.113) -> (15.5708, 51.8197) centre (15.5101, 51.9664) ccw
  arc A1926 (11.7811, 52.0763) -> (11.7811, 52.3938) centre (11.7811, 52.2351) ccw
  arc A1927 (13.6796, 52.0884) -> (13.5581, 52.3818) centre (13.6189, 52.2351) ccw
  arc A1928 (19.1689, 51.8223) -> (19.1689, 52.1398) centre (19.1689, 51.9811) ccw
  arc A1929 (12.5422, 52.0786) -> (12.3177, 51.8541) centre (12.4299, 51.9664) ccw
  arc A1930 (17.6222, 52.0786) -> (17.3977, 51.8541) centre (17.5099, 51.9664) ccw
  line L597 (17.9596, 51.5167) -> (17.51, 51.9663)
  arc A1931 (6.3546, 45.2309) -> (6.0612, 45.3524) centre (6.2079, 45.2917) ccw
  line L598 (10.4521, 47.0845) -> (10.4521, 46.1251)
  arc A1932 (9.1447, 46.0826) -> (9.0232, 45.7892) centre (9.084, 45.9359) ccw
  arc A1933 (18.1777, 51.5103) -> (17.9532, 51.7348) centre (18.0654, 51.6226) ccw
  arc A1934 (5.8229, 44.1544) -> (6.1405, 44.1544) centre (5.9817, 44.1544) ccw
  arc A1935 (9.084, 45.7771) -> (9.084, 46.0946) centre (9.084, 45.9359) ccw
  arc A1936 (17.8473, 51.629) -> (18.0719, 51.4044) centre (17.9596, 51.5167) ccw
  arc A1937 (9.7212, 45.6186) -> (9.9457, 45.3941) centre (9.8334, 45.5063) ccw
  arc A1938 (17.8473, 51.4044) -> (18.0719, 51.629) centre (17.9596, 51.5167) ccw
  arc A1939 (9.0232, 40.5708) -> (9.1447, 40.2774) centre (9.084, 40.4241) ccw
  arc A1940 (6.1405, 42.2056) -> (5.8229, 42.2056) centre (5.9817, 42.2056) ccw
  arc A1941 (9.7212, 45.3941) -> (9.9457, 45.6186) centre (9.8334, 45.5063) ccw
  line L599 (10.4521, 46.1251) -> (9.8334, 45.5064)
  line L600 (13.6189, 52.2351) -> (12.97, 51.9663)
  line L601 (7.172, 40.4241) -> (9.084, 40.4241)
  line L602 (6.6259, 45.7097) -> (6.2079, 45.2917)
  line L603 (5.9817, 44.7456) -> (5.9817, 44.1544)
  arc A1942 (6.5901, 43.0333) -> (6.7116, 43.3267) centre (6.6508, 43.18) ccw
  line L604 (6.6259, 43.1903) -> (6.6508, 43.18)
  arc A1943 (6.0957, 45.4039) -> (6.3202, 45.1794) centre (6.208, 45.2917) ccw
  line L605 (9.6301, 45.7097) -> (9.084, 45.9359)
  arc A1944 (10.3693, 52.113) -> (10.4908, 51.8197) centre (10.4301, 51.9664) ccw
  line L606 (15.51, 51.9663) -> (15.24, 51.6963)
  arc A1945 (6.5652, 45.8563) -> (6.6867, 45.563) centre (6.626, 45.7097) ccw
  line L607 (7.172, 45.9359) -> (6.6259, 45.7097)
  arc A1946 (6.3202, 41.1806) -> (6.0957, 40.956) centre (6.208, 41.0683) ccw
  line L608 (9.084, 45.9359) -> (7.172, 45.9359)
  arc A1947 (6.7116, 43.0333) -> (6.5901, 43.3267) centre (6.6508, 43.18) ccw
  arc A1948 (12.5877, 51.8086) -> (12.8123, 51.5841) centre (12.7, 51.6963) ccw
  line L609 (16.1589, 52.2351) -> (15.51, 51.9663)
  arc A1949 (6.5136, 43.0781) -> (6.7382, 43.3026) centre (6.6259, 43.1904) ccw
  line L610 (9.8334, 45.5064) -> (9.6301, 45.7097)
  line L611 (6.2079, 45.2917) -> (5.9817, 44.7456)
  arc A1950 (9.5693, 45.563) -> (9.6908, 45.8563) centre (9.6301, 45.7097) ccw
  arc A1951 (5.835, 44.8063) -> (6.1284, 44.6848) centre (5.9817, 44.7456) ccw
  arc A1952 (6.1284, 44.2152) -> (5.835, 44.0937) centre (5.9817, 44.1544) ccw
  arc A1953 (14.3819, 52.3818) -> (14.2604, 52.0884) centre (14.3211, 52.2351) ccw
  arc A1954 (15.0822, 52.0786) -> (14.8577, 51.8541) centre (14.9699, 51.9664) ccw
  arc A1955 (15.1277, 51.8086) -> (15.3523, 51.5841) centre (15.24, 51.6963) ccw
  line L612 (11.0789, 52.2351) -> (10.43, 51.9663)
  arc A1956 (7.2328, 45.7892) -> (7.1113, 46.0826) centre (7.1721, 45.9359) ccw
  arc A1957 (6.0612, 43.5476) -> (6.3546, 43.6691) centre (6.2079, 43.6084) ccw
  line L613 (6.6259, 43.1697) -> (6.2079, 42.7517)
  line L614 (6.6508, 43.18) -> (6.6259, 43.1697)
  arc A1958 (9.6908, 40.5036) -> (9.5693, 40.797) centre (9.6301, 40.6503) ccw
  arc A1959 (11.0789, 52.3938) -> (11.0789, 52.0763) centre (11.0789, 52.2351) ccw
  line L615 (9.084, 40.4241) -> (9.6301, 40.6503)
  arc A1960 (6.3202, 43.7206) -> (6.0957, 43.496) centre (6.2079, 43.6083) ccw
  line L616 (5.9817, 44.1544) -> (6.2079, 43.6083)
  arc A1961 (9.084, 40.2654) -> (9.084, 40.5829) centre (9.084, 40.4241) ccw
  line L617 (5.9817, 42.2056) -> (5.9817, 41.6144)
  arc A1962 (6.6867, 40.797) -> (6.5652, 40.5036) centre (6.626, 40.6503) ccw
  line L618 (14.3211, 52.2351) -> (13.6189, 52.2351)
  arc A1963 (7.172, 40.5829) -> (7.172, 40.2654) centre (7.172, 40.4241) ccw
  arc A1964 (10.4908, 47.2403) -> (10.3693, 46.947) centre (10.43, 47.0936) ccw
  line L619 (12.97, 51.9663) -> (12.7, 51.6963)
  arc A1965 (12.9093, 52.113) -> (13.0308, 51.8197) centre (12.9701, 51.9664) ccw
  line L620 (12.43, 51.9663) -> (11.7811, 52.2351)
  arc A1966 (14.9092, 51.8197) -> (15.0307, 52.113) centre (14.97, 51.9663) ccw
  arc A1967 (12.5877, 51.5841) -> (12.8123, 51.8086) centre (12.7, 51.6964) ccw
  arc A1968 (10.5644, 46.0128) -> (10.3398, 46.2373) centre (10.4521, 46.1251) ccw
  arc A1969 (7.172, 46.0946) -> (7.172, 45.7771) centre (7.172, 45.9359) ccw
  line L621 (11.7811, 52.2351) -> (11.0789, 52.2351)
  arc A1970 (14.2402, 42.552) -> (14.3617, 42.2586) centre (14.3009, 42.4053) ccw
  line L622 (6.6259, 35.5497) -> (6.3441, 35.2679)
  arc A1971 (15.746, 44.0556) -> (15.5214, 43.8311) centre (15.6337, 43.9434) ccw
  line L623 (10.7139, 41.081) -> (12.6596, 43.0266)
  arc A1972 (9.9358, 35.0194) -> (10.1603, 35.2439) centre (10.0481, 35.1317) ccw
  arc A1973 (7.1113, 40.2774) -> (7.2328, 40.5708) centre (7.1721, 40.4241) ccw
  arc A1974 (6.5652, 43.3164) -> (6.6866, 43.023) centre (6.6259, 43.1697) ccw
  arc A1975 (6.7382, 45.5974) -> (6.5136, 45.8219) centre (6.6259, 45.7097) ccw
  arc A1976 (9.7423, 45.8219) -> (9.5178, 45.5974) centre (9.63, 45.7097) ccw
  arc A1977 (10.6108, 47.0845) -> (10.2934, 47.0845) centre (10.4521, 47.0845) ccw
  arc A1978 (9.1447, 35.9226) -> (9.0232, 35.6292) centre (9.084, 35.7759) ccw
  arc A1979 (14.8002, 42.7708) -> (15.0247, 42.5463) centre (14.9124, 42.6586) ccw
  arc A1980 (5.835, 42.2663) -> (6.1284, 42.1448) centre (5.9817, 42.2056) ccw
  line L624 (13.4861, 31.4579) -> (10.2148, 34.7291)
  arc A1981 (6.6867, 43.337) -> (6.5651, 43.0437) centre (6.6259, 43.1904) ccw
  line L625 (13.6391, 42.4053) -> (14.3009, 42.4053)
  arc A1982 (9.5693, 35.403) -> (9.6908, 35.6963) centre (9.6301, 35.5496) ccw
  arc A1983 (15.8984, 32.2968) -> (15.6738, 32.5213) centre (15.7861, 32.409) ccw
  line L626 (6.2079, 43.6083) -> (6.6259, 43.1903)
  arc A1984 (14.8349, 31.2991) -> (14.8349, 31.6166) centre (14.8349, 31.4579) ccw
  arc A1985 (6.3546, 42.6909) -> (6.0612, 42.8124) centre (6.2079, 42.7516) ccw
  arc A1986 (9.9119, 41.0909) -> (9.9119, 40.7734) centre (9.9119, 40.9322) ccw
  arc A1987 (6.1405, 44.7456) -> (5.8229, 44.7456) centre (5.9817, 44.7456) ccw
  arc A1988 (6.1284, 41.6752) -> (5.835, 41.5537) centre (5.9817, 41.6144) ccw
  line L627 (9.6301, 35.5497) -> (9.084, 35.7759)
  line L628 (13.0276, 42.6586) -> (13.6391, 42.4053)
  line L629 (5.9817, 41.6144) -> (6.2079, 41.0683)
  line L630 (15.6337, 43.7381) -> (15.6337, 43.9433)
  line L631 (15.7861, 32.4091) -> (14.8349, 31.4579)
  line L632 (9.6301, 40.6503) -> (9.9119, 40.9321)
  line L633 (10.2148, 34.7291) -> (10.0481, 35.1317)
  arc A1989 (6.0957, 42.8639) -> (6.3202, 42.6394) centre (6.208, 42.7517) ccw
  arc A1990 (10.1947, 35.1924) -> (9.9014, 35.0709) centre (10.0481, 35.1317) ccw
  line L634 (9.084, 35.7759) -> (7.172, 35.7759)
  line L635 (6.6259, 40.6503) -> (7.172, 40.4241)
  arc A1991 (7.172, 35.9346) -> (7.172, 35.6171) centre (7.172, 35.7759) ccw
  line L636 (15.3804, 43.1266) -> (15.6337, 43.7381)
  arc A1992 (6.5652, 35.6963) -> (6.6867, 35.403) centre (6.626, 35.5496) ccw
  arc A1993 (6.0612, 41.0076) -> (6.3546, 41.1291) centre (6.2079, 41.0684) ccw
  arc A1994 (10.2934, 46.1251) -> (10.6108, 46.1251) centre (10.4521, 46.1251) ccw
  arc A1995 (10.6017, 41.1932) -> (10.8262, 40.9687) centre (10.714, 41.081) ccw
  arc A1996 (13.6391, 42.5641) -> (13.6391, 42.2466) centre (13.6391, 42.4054) ccw
  arc A1997 (6.5136, 40.5381) -> (6.7382, 40.7626) centre (6.6259, 40.6504) ccw
  line L637 (6.2079, 41.0683) -> (6.6259, 40.6503)
  arc A1998 (6.7382, 43.0574) -> (6.5136, 43.2819) centre (6.6259, 43.1696) ccw
  arc A1999 (10.3545, 40.7734) -> (10.3545, 41.0909) centre (10.3545, 40.9322) ccw
  arc A2000 (14.7227, 31.5702) -> (14.9472, 31.3456) centre (14.8349, 31.4579) ccw
  arc A2001 (13.4861, 31.6166) -> (13.4861, 31.2991) centre (13.4861, 31.4579) ccw
  arc A2002 (12.7718, 42.9144) -> (12.5473, 43.1389) centre (12.6596, 43.0267) ccw
  arc A2003 (15.4927, 43.0143) -> (15.2682, 43.2388) centre (15.3804, 43.1265) ccw
  arc A2004 (5.8229, 41.6144) -> (6.1405, 41.6144) centre (5.9817, 41.6144) ccw
  line L638 (7.172, 35.7759) -> (6.6259, 35.5497)
  arc A2005 (14.9732, 42.5119) -> (14.8517, 42.8052) centre (14.9125, 42.6586) ccw
  line L639 (6.2079, 42.7517) -> (5.9817, 42.2056)
  arc A2006 (9.084, 35.6171) -> (9.084, 35.9346) centre (9.084, 35.7759) ccw
  arc A2007 (7.2328, 35.6292) -> (7.1113, 35.9226) centre (7.172, 35.7759) ccw
  arc A2008 (13.0883, 42.8052) -> (12.9668, 42.5119) centre (13.0276, 42.6586) ccw
  arc A2009 (15.6738, 43.6787) -> (15.8984, 43.9032) centre (15.7861, 43.7909) ccw
  arc A2010 (15.7924, 43.9433) -> (15.4749, 43.9433) centre (15.6337, 43.9433) ccw
  arc A2011 (10.2938, 41.0788) -> (10.4153, 40.7854) centre (10.3546, 40.9321) ccw
  line L640 (21.8221, 44.4397) -> (21.276, 44.6659)
  line L641 (9.9119, 40.9321) -> (10.3545, 40.9321)
  arc A2012 (9.7423, 35.6619) -> (9.5178, 35.4374) centre (9.6301, 35.5496) ccw
  arc A2013 (22.3867, 44.0824) -> (22.0934, 43.9609) centre (22.2401, 44.0217) ccw
  line L642 (10.0481, 35.1317) -> (9.6301, 35.5497)
  line L643 (15.6337, 43.9433) -> (15.7861, 43.7909)
  arc A2014 (10.0682, 34.6684) -> (10.3615, 34.7899) centre (10.2149, 34.7292) ccw
  line L644 (14.8349, 31.4579) -> (13.4861, 31.4579)
  line L645 (10.3545, 40.9321) -> (10.7139, 41.081)
  arc A2015 (15.4749, 43.7381) -> (15.7924, 43.7381) centre (15.6337, 43.7381) ccw
  line L646 (14.9124, 42.6586) -> (15.3804, 43.1266)
  arc A2016 (14.3009, 42.2466) -> (14.3009, 42.5641) centre (14.3009, 42.4054) ccw
  arc A2017 (21.7613, 44.293) -> (21.8828, 44.5863) centre (21.8221, 44.4397) ccw
  arc A2018 (28.3146, 42.5255) -> (27.9971, 42.5255) centre (28.1559, 42.5255) ccw
  arc A2019 (25.3429, 42.5255) -> (25.0253, 42.5255) centre (25.1841, 42.5255) ccw
  line L647 (12.6596, 43.0266) -> (13.0276, 42.6586)
  arc A2020 (21.7364, 42.0567) -> (21.8579, 41.7633) centre (21.7972, 41.91) ccw
  line L648 (21.276, 44.6659) -> (19.364, 44.6659)
  arc A2021 (25.0718, 42.6377) -> (25.2964, 42.4132) centre (25.1841, 42.5255) ccw
  arc A2022 (10.3271, 34.8414) -> (10.1026, 34.6169) centre (10.2149, 34.7292) ccw
  line L649 (22.1039, 41.6179) -> (21.8221, 41.8997)
  arc A2023 (22.3196, 43.4148) -> (22.613, 43.5363) centre (22.4663, 43.4755) ccw
  line L650 (14.3009, 42.4053) -> (14.9124, 42.6586)
  arc A2024 (21.276, 44.5071) -> (21.276, 44.8246) centre (21.276, 44.6658) ccw
  arc A2025 (15.6274, 32.4091) -> (15.9449, 32.4091) centre (15.7862, 32.4091) ccw
  line L651 (15.7861, 43.7909) -> (15.7861, 32.4091)
  arc A2026 (13.3738, 31.3456) -> (13.5983, 31.5702) centre (13.4861, 31.4579) ccw
  arc A2027 (9.5178, 40.7626) -> (9.7423, 40.5381) centre (9.63, 40.6504) ccw
  arc A2028 (25.0253, 41.8071) -> (25.3429, 41.8071) centre (25.1841, 41.8071) ccw
  arc A2029 (21.7098, 42.0326) -> (21.9343, 41.8081) centre (21.8221, 41.9204) ccw
  line L652 (4.8319, 35.2679) -> (4.5501, 35.5497)
  arc A2030 (12.7718, 43.1389) -> (12.5473, 42.9144) centre (12.6595, 43.0267) ccw
  arc A2031 (21.9343, 42.0119) -> (21.7098, 41.7874) centre (21.8221, 41.8997) ccw
  arc A2032 (10.7747, 40.9343) -> (10.6532, 41.2276) centre (10.7139, 41.081) ccw
  line L653 (22.4663, 42.8844) -> (22.4663, 43.4756)
  arc A2033 (10.0241, 40.8198) -> (9.7996, 41.0444) centre (9.9119, 40.9321) ccw
  line L654 (25.1841, 41.8071) -> (24.9949, 41.6179)
  arc A2034 (15.9449, 43.7909) -> (15.6274, 43.7909) centre (15.7862, 43.7909) ccw
  arc A2035 (6.7382, 35.4374) -> (6.5136, 35.6619) centre (6.6259, 35.5496) ccw
  arc A2036 (4.4893, 35.403) -> (4.6108, 35.6963) centre (4.5501, 35.5496) ccw
  arc A2037 (21.9916, 41.5056) -> (22.2161, 41.7301) centre (22.1038, 41.6179) ccw
  arc A2038 (21.9343, 44.5519) -> (21.7098, 44.3274) centre (21.822, 44.4397) ccw
  line L655 (22.2401, 44.0217) -> (21.8221, 44.4397)
  arc A2039 (19.364, 44.8246) -> (19.364, 44.5071) centre (19.364, 44.6658) ccw
  arc A2040 (13.5783, 42.2586) -> (13.6998, 42.552) centre (13.639, 42.4053) ccw
  arc A2041 (12.9153, 42.5463) -> (13.1398, 42.7708) centre (13.0275, 42.6586) ccw
  arc A2042 (15.7804, 43.6773) -> (15.487, 43.7988) centre (15.6337, 43.7381) ccw
  arc A2043 (4.6623, 35.6619) -> (4.4378, 35.4374) centre (4.55, 35.5497) ccw
  arc A2044 (6.2319, 35.3802) -> (6.4564, 35.1556) centre (6.3441, 35.2679) ccw
  line L656 (4.5501, 35.5497) -> (4.004, 35.7759)
  arc A2045 (15.2337, 43.1873) -> (15.5271, 43.0658) centre (15.3804, 43.1266) ccw
  arc A2046 (21.3367, 44.8126) -> (21.2152, 44.5192) centre (21.2759, 44.6659) ccw
  arc A2047 (4.7196, 35.1556) -> (4.9441, 35.3802) centre (4.8319, 35.2679) ccw
  arc A2048 (22.613, 42.8237) -> (22.3196, 42.9452) centre (22.4663, 42.8845) ccw
  arc A2049 (18.9302, 44.3274) -> (18.7056, 44.5519) centre (18.8179, 44.4396) ccw
  arc A2050 (18.7572, 44.5863) -> (18.8787, 44.293) centre (18.8179, 44.4397) ccw
  line L657 (28.1559, 42.5255) -> (27.2855, 43.3959)
  line L658 (25.1841, 42.5255) -> (25.1841, 41.8071)
  arc A2051 (21.8828, 41.7736) -> (21.7614, 42.067) centre (21.8221, 41.9203) ccw
  line L659 (27.2855, 43.3959) -> (26.0545, 43.3959)
  line L660 (6.3441, 35.2679) -> (4.8319, 35.2679)
  line L661 (21.8221, 41.8997) -> (21.7972, 41.91)
  arc A2052 (21.7613, 41.753) -> (21.8828, 42.0463) centre (21.8221, 41.8997) ccw
  arc A2053 (22.1039, 41.7766) -> (22.1039, 41.4591) centre (22.1039, 41.6179) ccw
  arc A2054 (22.3523, 42.226) -> (22.1278, 42.4506) centre (22.24, 42.3383) ccw
  line L662 (24.9949, 41.6179) -> (22.1039, 41.6179)
  arc A2055 (22.0934, 42.3991) -> (22.3867, 42.2776) centre (22.2401, 42.3383) ccw
  arc A2056 (28.0436, 42.4132) -> (28.2682, 42.6377) centre (28.1559, 42.5255) ccw
  arc A2057 (22.3075, 42.8844) -> (22.625, 42.8844) centre (22.4663, 42.8844) ccw
  arc A2058 (4.0647, 35.9226) -> (3.9432, 35.6292) centre (4.004, 35.7759) ccw
  arc A2059 (6.3441, 35.1091) -> (6.3441, 35.4266) centre (6.3441, 35.2678) ccw
  arc A2060 (18.5466, 41.4209) -> (18.2532, 41.5424) centre (18.3999, 41.4817) ccw